Autodesk Fusion 360 part; units mm, degrees
(part 10 of 14)
  arc A2922 (59.8678, 11.2776) -> (59.8678, 11.7856) centre (59.8678, 11.5316) ccw
  line L4390 (48.7934, 56.1848) -> (48.1838, 56.1848)
  line L4391 (62.1538, 11.5316) -> (62.6618, 11.5316)
  arc A2923 (62.4078, 11.1379) -> (62.4078, 11.9253) centre (62.4078, 11.5316) ccw
  arc A2924 (62.4078, 11.9253) -> (62.4078, 11.1379) centre (62.4078, 11.5316) ccw
  line L4392 (62.4078, 11.2776) -> (62.4078, 11.7856)
  arc A2925 (62.4078, 11.9253) -> (62.4078, 11.1379) centre (62.4078, 11.5316) ccw
  arc A2926 (48.26, 58.6184) -> (48.26, 58.5168) centre (48.26, 58.5676) ccw
  line L4393 (48.9712, 60.833) -> (48.006, 60.833)
  arc A2927 (62.1602, 11.5316) -> (62.6555, 11.5316) centre (62.4078, 11.5316) ccw
  line L4394 (48.26, 58.5676) -> (48.768, 58.5676)
  line L4395 (48.1838, 57.2008) -> (48.7934, 57.2008)
  line L4396 (48.1838, 56.1848) -> (48.1838, 57.2008)
  line L4397 (48.7934, 56.1848) -> (48.1838, 56.1848)
  arc A2928 (59.8678, 11.7856) -> (59.8678, 11.2776) centre (59.8678, 11.5316) ccw
  line L4398 (62.4078, 11.2776) -> (62.4078, 11.7856)
  line L4399 (48.9712, 59.1566) -> (48.9712, 60.833)
  line L4400 (48.1838, 56.1848) -> (48.1838, 57.2008)
  arc A2929 (62.4078, 11.9253) -> (62.4078, 11.1379) centre (62.4078, 11.5316) ccw
  line L4401 (48.9386, 60.6948) -> (48.0386, 60.6948)
  arc A2930 (48.26, 58.5168) -> (48.26, 58.6184) centre (48.26, 58.5676) ccw
  arc A2931 (59.8678, 11.9253) -> (59.8678, 11.1379) centre (59.8678, 11.5316) ccw
  line L4402 (77.1398, 33.401) -> (76.5302, 33.401)
  arc A2932 (48.768, 58.0088) -> (48.768, 58.1104) centre (48.768, 58.0596) ccw
  line L4403 (48.9386, 60.6948) -> (48.0386, 60.6948)
  line L4404 (48.768, 58.0596) -> (48.26, 58.0596)
  line L4405 (76.2508, 33.784) -> (76.2508, 34.034)
  line L4406 (75.646, 34.459) -> (75.646, 33.359)
  line L4407 (48.9712, 60.833) -> (48.006, 60.833)
  line L4408 (41.36, 55.926) -> (41.36, 55.326)
  line L4409 (41.402, 55.3212) -> (41.402, 55.9308)
  line L4410 (76.2508, 34.034) -> (75.6412, 34.034)
  line L4411 (42.46, 55.326) -> (42.46, 55.926)
  line L4412 (75.6412, 34.034) -> (75.6412, 33.784)
  line L4413 (41.785, 60.5028) -> (41.785, 59.8932)
  line L4414 (48.9712, 59.1566) -> (48.9712, 60.833)
  line L4415 (76.5302, 34.417) -> (77.1398, 34.417)
  line L4416 (75.6412, 34.417) -> (76.2508, 34.417)
  arc A2933 (48.514, 58.0088) -> (48.514, 58.1104) centre (48.514, 58.0596) ccw
  line L4417 (77.135, 33.359) -> (77.135, 34.459)
  line L4418 (48.7934, 57.2008) -> (48.7934, 56.1848)
  line L4419 (48.514, 58.0596) -> (48.26, 58.5676)
  line L4420 (75.646, 33.359) -> (76.246, 33.359)
  line L4421 (76.535, 34.459) -> (76.535, 33.359)
  line L4422 (75.6412, 33.784) -> (76.2508, 33.784)
  line L4423 (75.6412, 33.401) -> (75.6412, 34.417)
  line L4424 (77.1398, 34.417) -> (77.1398, 33.401)
  line L4425 (77.1398, 33.401) -> (76.5302, 33.401)
  line L4426 (41.402, 60.5028) -> (42.418, 60.5028)
  line L4427 (42.035, 60.5028) -> (41.785, 60.5028)
  line L4428 (42.46, 59.898) -> (42.46, 60.498)
  line L4429 (42.418, 59.8932) -> (41.402, 59.8932)
  line L4430 (48.006, 59.1566) -> (48.9712, 59.1566)
  line L4431 (48.7886, 56.1428) -> (48.7886, 57.2428)
  line L4432 (48.1886, 57.2428) -> (48.1886, 56.1428)
  line L4433 (48.7934, 57.2008) -> (48.7934, 56.1848)
  arc A2934 (48.514, 58.1104) -> (48.514, 58.0088) centre (48.514, 58.0596) ccw
  line L4434 (76.5302, 33.784) -> (77.1398, 33.784)
  line L4435 (76.535, 33.359) -> (77.135, 33.359)
  line L4436 (76.246, 33.359) -> (76.246, 34.459)
  line L4437 (42.418, 60.5028) -> (42.418, 59.8932)
  line L4438 (42.418, 55.9308) -> (42.418, 55.3212)
  line L4439 (41.402, 59.8932) -> (41.402, 60.5028)
  line L4440 (41.402, 60.5028) -> (42.418, 60.5028)
  line L4441 (48.7886, 57.2428) -> (48.1886, 57.2428)
  line L4442 (76.2508, 33.401) -> (75.6412, 33.401)
  arc A2935 (48.768, 58.5168) -> (48.768, 58.6184) centre (48.768, 58.5676) ccw
  line L4443 (42.418, 59.8932) -> (41.402, 59.8932)
  line L4444 (48.9386, 59.2948) -> (48.0386, 59.2948)
  arc A2936 (48.768, 58.1104) -> (48.768, 58.0088) centre (48.768, 58.0596) ccw
  line L4445 (76.2508, 34.417) -> (76.2508, 33.401)
  line L4446 (76.5302, 33.401) -> (76.5302, 34.417)
  line L4447 (48.7934, 56.8178) -> (48.1838, 56.8178)
  line L4448 (76.246, 34.459) -> (75.646, 34.459)
  line L4449 (76.2508, 33.401) -> (75.6412, 33.401)
  line L4450 (41.402, 55.3212) -> (41.402, 55.9308)
  line L4451 (41.36, 55.326) -> (42.46, 55.326)
  line L4452 (41.785, 59.8932) -> (42.035, 59.8932)
  line L4453 (48.768, 58.5676) -> (48.514, 58.0596)
  line L4454 (75.6412, 33.401) -> (75.6412, 34.417)
  line L4455 (42.418, 55.3212) -> (41.402, 55.3212)
  line L4456 (77.135, 34.459) -> (76.535, 34.459)
  arc A2937 (48.768, 58.6184) -> (48.768, 58.5168) centre (48.768, 58.5676) ccw
  line L4457 (76.5302, 34.417) -> (77.1398, 34.417)
  line L4458 (41.785, 55.3212) -> (42.035, 55.3212)
  line L4459 (42.46, 55.926) -> (41.36, 55.926)
  line L4460 (74.041, 34.5948) -> (74.041, 33.9852)
  line L4461 (74.041, 34.8742) -> (73.025, 34.8742)
  line L4462 (73.025, 34.5948) -> (74.041, 34.5948)
  line L4463 (72.983, 34.879) -> (74.083, 34.879)
  line L4464 (73.658, 34.8742) -> (73.658, 35.4838)
  line L4465 (77.2668, 19.304) -> (76.6572, 19.304)
  line L4466 (76.6572, 19.937) -> (76.6572, 19.687)
  line L4467 (77.262, 20.362) -> (76.662, 20.362)
  line L4468 (74.083, 35.479) -> (72.983, 35.479)
  line L4469 (42.035, 59.8932) -> (42.035, 60.5028)
  line L4470 (74.041, 33.9852) -> (73.025, 33.9852)
  line L4471 (74.083, 34.879) -> (74.083, 35.479)
  line L4472 (72.983, 34.59) -> (72.983, 33.99)
  line L4473 (73.658, 34.5948) -> (73.408, 34.5948)
  line L4474 (73.408, 33.9852) -> (73.658, 33.9852)
  line L4475 (77.262, 19.262) -> (77.262, 20.362)
  line L4476 (76.5302, 33.401) -> (76.5302, 34.417)
  line L4477 (76.6572, 19.304) -> (76.6572, 20.32)
  line L4478 (73.025, 33.9852) -> (73.025, 34.5948)
  line L4479 (74.041, 34.8742) -> (73.025, 34.8742)
  line L4480 (74.083, 33.99) -> (74.083, 34.59)
  line L4481 (73.025, 35.4838) -> (74.041, 35.4838)
  line L4482 (73.025, 35.4838) -> (74.041, 35.4838)
  line L4483 (74.083, 34.59) -> (72.983, 34.59)
  line L4484 (73.408, 34.5948) -> (73.408, 33.9852)
  line L4485 (77.2668, 19.937) -> (76.6572, 19.937)
  line L4486 (76.6572, 19.304) -> (76.6572, 20.32)
  line L4487 (74.041, 34.5948) -> (74.041, 33.9852)
  line L4488 (76.6572, 20.32) -> (77.2668, 20.32)
  line L4489 (73.408, 35.4838) -> (73.408, 34.8742)
  line L4490 (76.662, 19.262) -> (77.262, 19.262)
  line L4491 (74.041, 33.9852) -> (73.025, 33.9852)
  line L4492 (74.041, 35.4838) -> (74.041, 34.8742)
  line L4493 (76.6572, 20.32) -> (77.2668, 20.32)
  line L4494 (75.6412, 34.417) -> (76.2508, 34.417)
  line L4495 (76.662, 20.362) -> (76.662, 19.262)
  line L4496 (76.5302, 34.034) -> (76.5302, 33.784)
  line L4497 (74.041, 35.4838) -> (74.041, 34.8742)
  line L4498 (77.2668, 20.32) -> (77.2668, 19.304)
  line L4499 (77.1398, 33.784) -> (77.1398, 34.034)
  line L4500 (41.402, 55.9308) -> (42.418, 55.9308)
  line L4501 (77.1398, 34.034) -> (76.5302, 34.034)
  line L4502 (42.035, 55.3212) -> (42.035, 55.9308)
  line L4503 (42.418, 55.3212) -> (41.402, 55.3212)
  line L4504 (41.785, 55.9308) -> (41.785, 55.3212)
  line L4505 (73.025, 34.5948) -> (74.041, 34.5948)
  line L4506 (77.1398, 34.417) -> (77.1398, 33.401)
  line L4507 (73.408, 34.8742) -> (73.658, 34.8742)
  line L4508 (41.402, 59.8932) -> (41.402, 60.5028)
  line L4509 (73.025, 33.9852) -> (73.025, 34.5948)
  line L4510 (42.418, 55.9308) -> (42.418, 55.3212)
  line L4511 (42.035, 55.9308) -> (41.785, 55.9308)
  line L4512 (76.2508, 34.417) -> (76.2508, 33.401)
  line L4513 (77.2668, 19.687) -> (77.2668, 19.937)
  line L4514 (72.983, 33.99) -> (74.083, 33.99)
  line L4515 (73.658, 35.4838) -> (73.408, 35.4838)
  line L4516 (41.402, 55.9308) -> (42.418, 55.9308)
  line L4517 (73.025, 34.8742) -> (73.025, 35.4838)
  line L4518 (72.983, 35.479) -> (72.983, 34.879)
  line L4519 (76.6572, 19.687) -> (77.2668, 19.687)
  line L4520 (77.2668, 19.304) -> (76.6572, 19.304)
  line L4521 (77.2668, 20.32) -> (77.2668, 19.304)
  line L4522 (73.658, 33.9852) -> (73.658, 34.5948)
  line L4523 (73.025, 34.8742) -> (73.025, 35.4838)
  line L4524 (61.849, 59.309) -> (61.849, 61.849)
  line L4525 (73.025, 19.2278) -> (74.041, 19.2278)
  line L4526 (59.5884, 59.5884) -> (61.5696, 59.5884)
  line L4527 (61.5696, 59.5884) -> (61.5696, 61.5696)
  line L4528 (76.3778, 20.32) -> (76.3778, 19.304)
  line L4529 (72.983, 19.512) -> (74.083, 19.512)
  line L4530 (75.7682, 20.32) -> (76.3778, 20.32)
  line L4531 (61.849, 61.849) -> (59.309, 61.849)
  line L4532 (73.408, 20.1168) -> (73.408, 19.5072)
  line L4533 (75.773, 20.362) -> (75.773, 19.262)
  line L4534 (74.041, 18.6182) -> (73.025, 18.6182)
  line L4535 (73.408, 18.6182) -> (73.658, 18.6182)
  line L4536 (72.983, 19.223) -> (72.983, 18.623)
  line L4537 (73.658, 18.6182) -> (73.658, 19.2278)
  line L4538 (76.373, 20.362) -> (75.773, 20.362)
  line L4539 (74.083, 20.112) -> (72.983, 20.112)
  line L4540 (73.025, 20.1168) -> (74.041, 20.1168)
  line L4541 (59.309, 59.944) -> (59.944, 59.309)
  line L4542 (59.944, 59.309) -> (61.849, 59.309)
  line L4543 (59.5884, 61.5696) -> (59.5884, 59.5884)
  line L4544 (66.3956, 61.5696) -> (64.4144, 61.5696)
  line L4545 (73.025, 18.6182) -> (73.025, 19.2278)
  line L4546 (72.983, 20.112) -> (72.983, 19.512)
  line L4547 (75.773, 19.262) -> (76.373, 19.262)
  line L4548 (74.041, 20.1168) -> (74.041, 19.5072)
  line L4549 (75.7682, 20.32) -> (76.3778, 20.32)
  line L4550 (62.0776, 59.4741) -> (62.0776, 61.6839)
  line L4551 (66.675, 61.849) -> (64.135, 61.849)
  line L4552 (66.675, 59.309) -> (66.675, 61.849)
  line L4553 (59.0804, 59.4741) -> (59.0804, 61.6839)
  line L4554 (64.135, 61.849) -> (64.135, 59.944)
  line L4555 (73.658, 19.5072) -> (73.658, 20.1168)
  line L4556 (74.083, 19.223) -> (72.983, 19.223)
  line L4557 (75.7682, 19.304) -> (75.7682, 20.32)
  line L4558 (73.658, 20.1168) -> (73.408, 20.1168)
  line L4559 (72.983, 18.623) -> (74.083, 18.623)
  line L4560 (76.3778, 19.687) -> (76.3778, 19.937)
  line L4561 (75.7682, 19.304) -> (75.7682, 20.32)
  line L4562 (62.0776, 59.4741) -> (62.0776, 61.6839)
  line L4563 (59.309, 61.849) -> (59.309, 59.944)
  line L4564 (75.7682, 19.937) -> (75.7682, 19.687)
  line L4565 (73.408, 19.2278) -> (73.408, 18.6182)
  line L4566 (74.083, 19.512) -> (74.083, 20.112)
  line L4567 (76.373, 19.262) -> (76.373, 20.362)
  line L4568 (73.025, 18.6182) -> (73.025, 19.2278)
  line L4569 (74.041, 20.1168) -> (74.041, 19.5072)
  line L4570 (74.041, 19.2278) -> (74.041, 18.6182)
  line L4571 (76.3778, 19.937) -> (75.7682, 19.937)
  line L4572 (75.7682, 19.687) -> (76.3778, 19.687)
  line L4573 (74.041, 19.5072) -> (73.025, 19.5072)
  line L4574 (73.658, 19.2278) -> (73.408, 19.2278)
  line L4575 (73.025, 19.5072) -> (73.025, 20.1168)
  line L4576 (74.041, 19.2278) -> (74.041, 18.6182)
  line L4577 (76.3778, 19.304) -> (75.7682, 19.304)
  line L4578 (61.5696, 61.5696) -> (59.5884, 61.5696)
  line L4579 (76.3778, 20.32) -> (76.3778, 19.304)
  line L4580 (74.083, 18.623) -> (74.083, 19.223)
  line L4581 (73.025, 20.1168) -> (74.041, 20.1168)
  line L4582 (73.025, 19.2278) -> (74.041, 19.2278)
  line L4583 (76.3778, 19.304) -> (75.7682, 19.304)
  line L4584 (74.041, 19.5072) -> (73.025, 19.5072)
  line L4585 (73.025, 19.5072) -> (73.025, 20.1168)
  line L4586 (74.041, 18.6182) -> (73.025, 18.6182)
  line L4587 (73.408, 19.5072) -> (73.658, 19.5072)
  line L4588 (84.917, 57.362) -> (85.517, 57.362)
  line L4589 (22.733, 53.1368) -> (22.733, 49.7332)
  line L4590 (85.517, 57.362) -> (85.517, 58.462)
  line L4591 (84.9122, 58.42) -> (85.5218, 58.42)
  line L4592 (26.455, 42.675) -> (28.155, 42.675)
  line L4593 (60.071, 59.0804) -> (61.087, 59.0804)
  line L4594 (66.9036, 59.4741) -> (66.9036, 61.6839)
  line L4595 (26.455, 39.875) -> (28.155, 39.875)
  line L4596 (28.205, 42.975) -> (26.405, 42.975)
  line L4597 (26.405, 39.575) -> (28.205, 39.575)
  line L4598 (60.071, 62.0776) -> (61.087, 62.0776)
  line L4599 (28.194, 42.9768) -> (26.416, 42.9768)
  line L4600 (84.9122, 58.42) -> (85.5218, 58.42)
  line L4601 (85.517, 58.462) -> (84.917, 58.462)
  line L4602 (28.194, 42.9768) -> (26.416, 42.9768)
  line L4603 (63.9064, 59.4741) -> (63.9064, 61.6839)
  line L4604 (26.416, 39.5732) -> (28.194, 39.5732)
  line L4605 (64.897, 62.0776) -> (65.913, 62.0776)
  line L4606 (63.9064, 59.4741) -> (63.9064, 61.6839)
  line L4607 (84.9122, 57.404) -> (84.9122, 58.42)
  line L4608 (24.522, 49.735) -> (24.522, 53.135)
  line L4609 (64.4144, 61.5696) -> (64.4144, 59.5884)
  line L4610 (66.9036, 59.4741) -> (66.9036, 61.6839)
  line L4611 (85.5218, 58.42) -> (85.5218, 57.404)
  line L4612 (28.194, 39.5732) -> (28.194, 42.9768)
  line L4613 (24.511, 49.7332) -> (24.511, 53.1368)
  line L4614 (22.722, 53.135) -> (22.722, 49.735)
  line L4615 (24.511, 53.1368) -> (22.733, 53.1368)
  line L4616 (60.071, 59.0804) -> (61.087, 59.0804)
  line L4617 (26.416, 42.9768) -> (26.416, 39.5732)
  line L4618 (85.5218, 58.037) -> (84.9122, 58.037)
  line L4619 (22.733, 53.1368) -> (22.733, 49.7332)
  line L4620 (22.733, 49.7332) -> (24.511, 49.7332)
  line L4621 (22.733, 49.7332) -> (24.511, 49.7332)
  line L4622 (84.9122, 57.404) -> (84.9122, 58.42)
  line L4623 (59.0804, 59.4741) -> (59.0804, 61.6839)
  line L4624 (66.9036, 59.4741) -> (66.9036, 61.6839)
  line L4625 (26.455, 42.675) -> (28.155, 42.675)
  line L4626 (22.722, 49.735) -> (24.522, 49.735)
  line L4627 (64.897, 59.0804) -> (65.913, 59.0804)
  line L4628 (64.897, 59.0804) -> (65.913, 59.0804)
  line L4629 (59.0804, 59.4741) -> (59.0804, 61.6839)
  line L4630 (64.897, 62.0776) -> (65.913, 62.0776)
  line L4631 (62.0776, 59.4741) -> (62.0776, 61.6839)
  line L4632 (60.071, 62.0776) -> (61.087, 62.0776)
  line L4633 (64.135, 59.944) -> (64.77, 59.309)
  line L4634 (66.3956, 59.5884) -> (66.3956, 61.5696)
  line L4635 (64.77, 59.309) -> (66.675, 59.309)
  line L4636 (60.071, 62.0776) -> (61.087, 62.0776)
  line L4637 (60.071, 59.0804) -> (61.087, 59.0804)
  line L4638 (64.4144, 59.5884) -> (66.3956, 59.5884)
  line L4639 (28.205, 39.575) -> (28.205, 42.975)
  line L4640 (64.897, 59.0804) -> (65.913, 59.0804)
  line L4641 (85.5218, 57.404) -> (84.9122, 57.404)
  line L4642 (84.9122, 57.787) -> (85.5218, 57.787)
  line L4643 (64.897, 62.0776) -> (65.913, 62.0776)
  line L4644 (28.194, 39.5732) -> (28.194, 42.9768)
  line L4645 (26.455, 39.875) -> (28.155, 39.875)
  line L4646 (84.9122, 58.037) -> (84.9122, 57.787)
  line L4647 (24.511, 49.7332) -> (24.511, 53.1368)
  line L4648 (85.5218, 58.42) -> (85.5218, 57.404)
  line L4649 (26.416, 42.9768) -> (26.416, 39.5732)
  line L4650 (63.9064, 59.4741) -> (63.9064, 61.6839)
  line L4651 (26.416, 39.5732) -> (28.194, 39.5732)
  line L4652 (74.589, 2.579) -> (73.239, 2.579)
  line L4653 (68.1482, 2.286) -> (68.1482, 4.572)
  line L4654 (22.772, 52.835) -> (24.472, 52.835)
  line L4655 (86.106, 52.1208) -> (86.106, 53.5432)
  line L4656 (83.863, 53.557) -> (83.863, 52.107)
  line L4657 (66.712, 4.529) -> (66.712, 2.329)
  line L4658 (24.511, 53.1368) -> (22.733, 53.1368)
  line L4659 (68.1482, 2.286) -> (68.1482, 4.572)
  line L4660 (86.106, 53.5432) -> (83.82, 53.5432)
  line L4661 (83.399, 56.095) -> (84.749, 56.095)
  line L4662 (83.399, 56.095) -> (84.749, 56.095)
  line L4663 (73.189, 4.529) -> (73.189, 2.329)
  line L4664 (83.82, 52.1208) -> (86.106, 52.1208)
  line L4665 (22.772, 52.835) -> (24.472, 52.835)
  line L4666 (66.762, 4.279) -> (68.112, 4.279)
  line L4667 (73.2028, 4.572) -> (73.2028, 2.286)
  line L4668 (66.762, 4.279) -> (68.112, 4.279)
  line L4669 (84.113, 53.507) -> (84.113, 52.157)
  line L4670 (22.772, 50.035) -> (24.472, 50.035)
  line L4671 (85.813, 53.507) -> (85.813, 52.157)
  line L4672 (66.762, 2.579) -> (68.112, 2.579)
  line L4673 (85.5218, 57.404) -> (84.9122, 57.404)
  line L4674 (66.712, 2.329) -> (68.162, 2.329)
  line L4675 (74.639, 2.329) -> (74.639, 4.529)
  line L4676 (22.772, 50.035) -> (24.472, 50.035)
  line L4677 (84.7852, 54.102) -> (84.7852, 56.388)
  line L4678 (86.063, 52.107) -> (86.063, 53.557)
  line L4679 (84.7852, 56.388) -> (83.3628, 56.388)
  line L4680 (68.162, 2.329) -> (68.162, 4.529)
  line L4681 (73.2028, 2.286) -> (74.6252, 2.286)
  line L4682 (66.7258, 2.286) -> (68.1482, 2.286)
  line L4683 (74.6252, 2.286) -> (74.6252, 4.572)
  line L4684 (83.82, 52.1208) -> (86.106, 52.1208)
  line L4685 (74.589, 2.579) -> (73.239, 2.579)
  line L4686 (66.7258, 2.286) -> (68.1482, 2.286)
  line L4687 (73.2028, 2.286) -> (74.6252, 2.286)
  line L4688 (68.1482, 4.572) -> (66.7258, 4.572)
  line L4689 (68.162, 4.529) -> (66.712, 4.529)
  line L4690 (66.762, 4.279) -> (68.112, 4.279)
  line L4691 (84.917, 58.462) -> (84.917, 57.362)
  line L4692 (26.405, 42.975) -> (26.405, 39.575)
  line L4693 (24.522, 53.135) -> (22.722, 53.135)
  line L4694 (74.639, 4.529) -> (73.189, 4.529)
  line L4695 (26.455, 42.675) -> (28.155, 42.675)
  line L4696 (66.7258, 4.572) -> (66.7258, 2.286)
  line L4697 (22.772, 50.035) -> (24.472, 50.035)
  line L4698 (66.7258, 4.572) -> (66.7258, 2.286)
  line L4699 (74.6252, 2.286) -> (74.6252, 4.572)
  line L4700 (74.6252, 4.572) -> (73.2028, 4.572)
  line L4701 (85.5218, 57.787) -> (85.5218, 58.037)
  line L4702 (68.1482, 4.572) -> (66.7258, 4.572)
  line L4703 (73.189, 2.329) -> (74.639, 2.329)
  line L4704 (26.455, 39.875) -> (28.155, 39.875)
  line L4705 (73.2028, 4.572) -> (73.2028, 2.286)
  line L4706 (66.762, 2.579) -> (68.112, 2.579)
  line L4707 (84.7852, 56.388) -> (83.3628, 56.388)
  line L4708 (83.399, 54.395) -> (84.749, 54.395)
  line L4709 (83.399, 54.395) -> (84.749, 54.395)
  line L4710 (74.6252, 4.572) -> (73.2028, 4.572)
  line L4711 (74.589, 4.279) -> (73.239, 4.279)
  line L4712 (22.772, 52.835) -> (24.472, 52.835)
  line L4713 (83.399, 54.395) -> (84.749, 54.395)
  line L4714 (66.762, 2.579) -> (68.112, 2.579)
  line L4715 (74.589, 2.579) -> (73.239, 2.579)
  line L4716 (27.85, 58.844) -> (29.3, 58.844)
  line L4717 (84.799, 54.145) -> (84.799, 56.345)
  line L4718 (83.399, 56.095) -> (84.749, 56.095)
  line L4719 (83.3628, 56.388) -> (83.3628, 54.102)
  line L4720 (32.385, 32.5628) -> (32.385, 33.9852)
  line L4721 (32.385, 33.9852) -> (30.099, 33.9852)
  line L4722 (83.863, 52.107) -> (86.063, 52.107)
  line L4723 (32.342, 36.666) -> (30.142, 36.666)
  line L4724 (32.342, 35.216) -> (32.342, 36.666)
  line L4725 (32.092, 33.949) -> (32.092, 32.599)
  line L4726 (83.3628, 56.388) -> (83.3628, 54.102)
  line L4727 (29.3, 61.044) -> (27.85, 61.044)
  line L4728 (84.113, 53.507) -> (84.113, 52.157)
  line L4729 (30.142, 35.216) -> (32.342, 35.216)
  line L4730 (27.8638, 58.801) -> (29.2862, 58.801)
  line L4731 (30.099, 33.9852) -> (30.099, 32.5628)
  line L4732 (83.349, 54.145) -> (84.799, 54.145)
  line L4733 (29.2862, 61.087) -> (27.8638, 61.087)
  line L4734 (74.589, 4.279) -> (73.239, 4.279)
  line L4735 (85.813, 53.507) -> (85.813, 52.157)
  line L4736 (30.099, 35.2298) -> (32.385, 35.2298)
  line L4737 (32.385, 36.6522) -> (30.099, 36.6522)
  line L4738 (32.092, 36.616) -> (32.092, 35.266)
  line L4739 (27.85, 61.044) -> (27.85, 58.844)
  line L4740 (29.3, 58.844) -> (29.3, 61.044)
  line L4741 (30.142, 36.666) -> (30.142, 35.216)
  line L4742 (30.099, 33.9852) -> (30.099, 32.5628)
  line L4743 (30.392, 33.949) -> (30.392, 32.599)
  line L4744 (84.799, 56.345) -> (83.349, 56.345)
  line L4745 (84.113, 53.507) -> (84.113, 52.157)
  line L4746 (85.813, 53.507) -> (85.813, 52.157)
  line L4747 (83.82, 53.5432) -> (83.82, 52.1208)
  line L4748 (32.342, 33.999) -> (30.142, 33.999)
  line L4749 (32.342, 32.549) -> (32.342, 33.999)
  line L4750 (32.385, 36.6522) -> (30.099, 36.6522)
  line L4751 (86.106, 53.5432) -> (83.82, 53.5432)
  line L4752 (30.392, 36.616) -> (30.392, 35.266)
  line L4753 (32.385, 32.5628) -> (32.385, 33.9852)
  line L4754 (86.063, 53.557) -> (83.863, 53.557)
  line L4755 (30.099, 32.5628) -> (32.385, 32.5628)
  line L4756 (83.82, 53.5432) -> (83.82, 52.1208)
  line L4757 (74.589, 4.279) -> (73.239, 4.279)
  line L4758 (30.099, 32.5628) -> (32.385, 32.5628)
  line L4759 (32.385, 33.9852) -> (30.099, 33.9852)
  line L4760 (84.7852, 54.102) -> (84.7852, 56.388)
  line L4761 (32.092, 36.616) -> (32.092, 35.266)
  line L4762 (27.8638, 61.087) -> (27.8638, 58.801)
  line L4763 (30.099, 35.2298) -> (32.385, 35.2298)
  line L4764 (32.092, 33.949) -> (32.092, 32.599)
  line L4765 (30.142, 32.549) -> (32.342, 32.549)
  line L4766 (30.392, 33.949) -> (30.392, 32.599)
  line L4767 (83.3628, 54.102) -> (84.7852, 54.102)
  line L4768 (27.8638, 61.087) -> (27.8638, 58.801)
  line L4769 (30.099, 36.6522) -> (30.099, 35.2298)
  line L4770 (30.392, 36.616) -> (30.392, 35.266)
  line L4771 (32.092, 36.616) -> (32.092, 35.266)
  line L4772 (86.106, 52.1208) -> (86.106, 53.5432)
  line L4773 (30.392, 33.949) -> (30.392, 32.599)
  line L4774 (30.392, 36.616) -> (30.392, 35.266)
  line L4775 (29.2862, 58.801) -> (29.2862, 61.087)
  line L4776 (83.3628, 54.102) -> (84.7852, 54.102)
  line L4777 (32.385, 35.2298) -> (32.385, 36.6522)
  line L4778 (83.349, 56.345) -> (83.349, 54.145)
  line L4779 (30.142, 33.999) -> (30.142, 32.549)
  line L4780 (32.092, 33.949) -> (32.092, 32.599)
  line L4781 (29.805, 61.81) -> (31.155, 61.81)
  line L4782 (29.7688, 59.817) -> (31.1912, 59.817)
  arc A2938 (64.897, 52.04) -> (64.897, 52.608) centre (64.897, 52.324) ccw
  line L4783 (66.3067, 54.098) -> (65.4177, 54.098)
  line L4784 (66.3067, 55.098) -> (65.4177, 55.098)
  line L4785 (29.7688, 59.817) -> (31.1912, 59.817)
  line L4786 (65.4558, 51.308) -> (60.833, 51.308)
  line L4787 (66.3067, 54.098) -> (65.4177, 54.098)
  line L4788 (66.3067, 55.598) -> (65.4177, 55.598)
  line L4789 (65.123, 55.8927) -> (65.123, 56.7817)
  line L4790 (31.205, 59.86) -> (31.205, 62.06)
  line L4791 (29.805, 60.11) -> (31.155, 60.11)
  line L4792 (31.1912, 62.103) -> (29.7688, 62.103)
  line L4793 (31.1912, 59.817) -> (31.1912, 62.103)
  line L4794 (66.3067, 55.598) -> (65.4177, 55.598)
  line L4795 (29.805, 60.11) -> (31.155, 60.11)
  line L4796 (66.3067, 52.098) -> (65.4177, 52.098)
  line L4797 (27.9, 60.794) -> (29.25, 60.794)
  line L4798 (66.3067, 52.098) -> (65.4177, 52.098)
  line L4799 (29.7688, 62.103) -> (29.7688, 59.817)
  line L4800 (66.3067, 54.598) -> (65.4177, 54.598)
  line L4801 (66.3067, 52.598) -> (65.4177, 52.598)
  line L4802 (66.3067, 54.098) -> (65.4177, 54.098)
  line L4803 (66.3067, 54.598) -> (65.4177, 54.598)
  line L4804 (66.3067, 54.598) -> (65.4177, 54.598)
  line L4805 (29.7688, 62.103) -> (29.7688, 59.817)
  line L4806 (66.3067, 53.598) -> (65.4177, 53.598)
  line L4807 (66.3067, 52.098) -> (65.4177, 52.098)
  line L4808 (60.833, 56.388) -> (65.913, 56.388)
  line L4809 (60.833, 51.308) -> (60.833, 56.388)
  line L4810 (27.8638, 58.801) -> (29.2862, 58.801)
  line L4811 (29.805, 60.11) -> (31.155, 60.11)
  line L4812 (65.913, 51.7652) -> (65.4558, 51.308)
  line L4813 (29.2862, 61.087) -> (27.8638, 61.087)
  line L4814 (31.205, 62.06) -> (29.755, 62.06)
  line L4815 (30.099, 36.6522) -> (30.099, 35.2298)
  line L4816 (27.9, 60.794) -> (29.25, 60.794)
  line L4817 (31.1912, 59.817) -> (31.1912, 62.103)
  line L4818 (27.9, 59.094) -> (29.25, 59.094)
  line L4819 (66.3067, 55.098) -> (65.4177, 55.098)
  line L4820 (66.3067, 52.598) -> (65.4177, 52.598)
  line L4821 (29.755, 59.86) -> (31.205, 59.86)
  line L4822 (32.385, 35.2298) -> (32.385, 36.6522)
  arc A2939 (64.897, 52.608) -> (64.897, 52.04) centre (64.897, 52.324) ccw
  line L4823 (65.913, 56.388) -> (65.913, 51.7652)
  arc A2940 (66.597, 51.808) -> (66.597, 51.24) centre (66.597, 51.524) ccw
  line L4824 (66.3067, 53.598) -> (65.4177, 53.598)
  line L4825 (66.3067, 52.598) -> (65.4177, 52.598)
  line L4826 (29.805, 61.81) -> (31.155, 61.81)
  line L4827 (31.1912, 62.103) -> (29.7688, 62.103)
  line L4828 (27.9, 59.094) -> (29.25, 59.094)
  line L4829 (66.3067, 55.098) -> (65.4177, 55.098)
  line L4830 (66.3067, 53.098) -> (65.4177, 53.098)
  line L4831 (27.9, 60.794) -> (29.25, 60.794)
  line L4832 (29.755, 62.06) -> (29.755, 59.86)
  arc A2941 (66.597, 51.24) -> (66.597, 51.808) centre (66.597, 51.524) ccw
  line L4833 (29.2862, 58.801) -> (29.2862, 61.087)
  line L4834 (29.805, 61.81) -> (31.155, 61.81)
  line L4835 (27.9, 59.094) -> (29.25, 59.094)
  line L4836 (66.3067, 53.098) -> (65.4177, 53.098)
  line L4837 (66.3067, 53.098) -> (65.4177, 53.098)
  line L4838 (66.3067, 55.598) -> (65.4177, 55.598)
  line L4839 (66.3067, 53.598) -> (65.4177, 53.598)
  line L4840 (21.9227, 8.9205) -> (21.9227, 9.5301)
  line L4841 (22.3058, 9.5301) -> (22.3058, 8.9205)
  line L4842 (63.373, 52.7488) -> (63.373, 55.0488)
  line L4843 (22.3058, 8.9205) -> (22.5557, 8.9205)
  line L4844 (22.5557, 9.5301) -> (22.3058, 9.5301)
  line L4845 (61.3283, 54.598) -> (60.4393, 54.598)
  line L4846 (21.9227, 9.5301) -> (22.9387, 9.5301)
  line L4847 (63.373, 52.7488) -> (63.373, 55.0488)
  line L4848 (22.5557, 8.9205) -> (22.5557, 9.5301)
  line L4849 (22.9807, 9.5253) -> (21.8807, 9.5253)
  line L4850 (61.3283, 53.598) -> (60.4393, 53.598)
  line L4851 (61.623, 50.9143) -> (61.623, 51.8033)
  line L4852 (61.3283, 52.598) -> (60.4393, 52.598)
  line L4853 (65.123, 50.9143) -> (65.123, 51.8033)
  line L4854 (63.123, 50.9143) -> (63.123, 51.8033)
  line L4855 (62.623, 50.9143) -> (62.623, 51.8033)
  line L4856 (61.3283, 53.098) -> (60.4393, 53.098)
  line L4857 (61.3283, 54.598) -> (60.4393, 54.598)
  line L4858 (61.623, 50.9143) -> (61.623, 51.8033)
  line L4859 (62.123, 50.9143) -> (62.123, 51.8033)
  line L4860 (65.123, 50.9143) -> (65.123, 51.8033)
  line L4861 (61.3283, 53.098) -> (60.4393, 53.098)
  line L4862 (61.3283, 53.598) -> (60.4393, 53.598)
  line L4863 (64.123, 50.9143) -> (64.123, 51.8033)
  line L4864 (64.123, 50.9143) -> (64.123, 51.8033)
  line L4865 (22.9387, 8.9205) -> (21.9227, 8.9205)
  line L4866 (61.3283, 52.598) -> (60.4393, 52.598)
  line L4867 (64.123, 50.9143) -> (64.123, 51.8033)
  line L4868 (64.623, 50.9143) -> (64.623, 51.8033)
  line L4869 (21.8807, 8.9253) -> (22.9807, 8.9253)
  line L4870 (61.623, 50.9143) -> (61.623, 51.8033)
  line L4871 (62.123, 50.9143) -> (62.123, 51.8033)
  line L4872 (21.9227, 8.9205) -> (21.9227, 9.5301)
  line L4873 (52.7558, 44.071) -> (52.7558, 44.321)
  line L4874 (63.123, 50.9143) -> (63.123, 51.8033)
  line L4875 (61.3283, 52.598) -> (60.4393, 52.598)
  line L4876 (54.2798, 45.339) -> (54.2798, 44.323)
  line L4877 (52.1462, 44.704) -> (52.7558, 44.704)
  line L4878 (61.3283, 54.098) -> (60.4393, 54.098)
  line L4879 (61.3283, 53.598) -> (60.4393, 53.598)
  line L4880 (63.623, 50.9143) -> (63.623, 51.8033)
  line L4881 (22.9387, 8.9205) -> (21.9227, 8.9205)
  line L4882 (63.123, 50.9143) -> (63.123, 51.8033)
  line L4883 (61.3283, 52.098) -> (60.4393, 52.098)
  line L4884 (61.3283, 54.098) -> (60.4393, 54.098)
  line L4885 (61.3283, 52.098) -> (60.4393, 52.098)
  line L4886 (62.123, 50.9143) -> (62.123, 51.8033)
  line L4887 (63.623, 50.9143) -> (63.623, 51.8033)
  line L4888 (63.623, 50.9143) -> (63.623, 51.8033)
  line L4889 (65.123, 50.9143) -> (65.123, 51.8033)
  line L4890 (63.373, 52.7488) -> (63.373, 55.0488)
  line L4891 (54.2798, 44.956) -> (53.6702, 44.956)
  line L4892 (62.623, 50.9143) -> (62.623, 51.8033)
  line L4893 (21.9227, 9.5301) -> (22.9387, 9.5301)
  line L4894 (64.623, 50.9143) -> (64.623, 51.8033)
  line L4895 (61.3283, 53.098) -> (60.4393, 53.098)
  line L4896 (61.3283, 54.098) -> (60.4393, 54.098)
  line L4897 (22.9807, 8.9253) -> (22.9807, 9.5253)
  line L4898 (64.623, 50.9143) -> (64.623, 51.8033)
  line L4899 (62.623, 50.9143) -> (62.623, 51.8033)
  line L4900 (21.8807, 9.5253) -> (21.8807, 8.9253)
  line L4901 (22.9387, 9.5301) -> (22.9387, 8.9205)
  line L4902 (22.9387, 9.5301) -> (22.9387, 8.9205)
  line L4903 (61.3283, 52.098) -> (60.4393, 52.098)
  line L4904 (60.625, 44.492) -> (60.025, 44.492)
  line L4905 (61.6458, 44.45) -> (61.6458, 43.434)
  line L4906 (61.0362, 43.434) -> (61.0362, 44.45)
  line L4907 (61.0362, 43.817) -> (61.6458, 43.817)
  line L4908 (60.025, 44.492) -> (60.025, 43.392)
  line L4909 (52.751, 44.746) -> (52.151, 44.746)
  line L4910 (60.0202, 43.817) -> (60.6298, 43.817)
  line L4911 (52.7558, 44.321) -> (52.1462, 44.321)
  line L4912 (53.675, 45.381) -> (53.675, 44.281)
  line L4913 (54.2798, 44.323) -> (53.6702, 44.323)
  line L4914 (60.6298, 44.067) -> (60.0202, 44.067)
  line L4915 (52.151, 44.746) -> (52.151, 43.646)
  line L4916 (54.2798, 44.323) -> (53.6702, 44.323)
  line L4917 (67.312, 54.4322) -> (67.562, 54.4322)
  line L4918 (61.041, 43.392) -> (61.641, 43.392)
  line L4919 (60.625, 43.392) -> (60.625, 44.492)
  line L4920 (61.0362, 44.45) -> (61.6458, 44.45)
  line L4921 (52.1462, 44.704) -> (52.7558, 44.704)
  line L4922 (53.6702, 44.956) -> (53.6702, 44.706)
  line L4923 (52.7558, 43.688) -> (52.1462, 43.688)
  line L4924 (68.495, 50.465) -> (67.395, 50.465)
  line L4925 (53.6702, 44.323) -> (53.6702, 45.339)
  line L4926 (52.1462, 43.688) -> (52.1462, 44.704)
  line L4927 (53.6702, 45.339) -> (54.2798, 45.339)
  line L4928 (54.275, 44.281) -> (54.275, 45.381)
  line L4929 (66.929, 54.4322) -> (66.929, 55.0418)
  line L4930 (64.9732, 49.657) -> (65.5828, 49.657)
  line L4931 (65.578, 48.599) -> (65.578, 49.699)
  line L4932 (52.7558, 44.704) -> (52.7558, 43.688)
  line L4933 (61.041, 44.492) -> (61.041, 43.392)
  line L4934 (67.562, 54.1528) -> (67.312, 54.1528)
  line L4935 (67.945, 54.1528) -> (67.945, 53.5432)
  line L4936 (66.929, 53.5432) -> (66.929, 54.1528)
  line L4937 (60.6298, 44.45) -> (60.6298, 43.434)
  line L4938 (66.929, 55.0418) -> (67.945, 55.0418)
  line L4939 (60.6298, 43.434) -> (60.0202, 43.434)
  line L4940 (60.0202, 43.434) -> (60.0202, 44.45)
  line L4941 (52.1462, 44.321) -> (52.1462, 44.071)
  line L4942 (54.275, 45.381) -> (53.675, 45.381)
  line L4943 (60.0202, 44.45) -> (60.6298, 44.45)
  line L4944 (53.6702, 44.706) -> (54.2798, 44.706)
  line L4945 (60.6298, 43.434) -> (60.0202, 43.434)
  line L4946 (60.0202, 44.067) -> (60.0202, 43.817)
  line L4947 (53.6702, 45.339) -> (54.2798, 45.339)
  line L4948 (53.6702, 44.323) -> (53.6702, 45.339)
  line L4949 (54.2798, 45.339) -> (54.2798, 44.323)
  line L4950 (60.6298, 43.817) -> (60.6298, 44.067)
  line L4951 (52.151, 43.646) -> (52.751, 43.646)
  line L4952 (61.6458, 44.45) -> (61.6458, 43.434)
  line L4953 (60.6298, 44.45) -> (60.6298, 43.434)
  line L4954 (61.641, 43.392) -> (61.641, 44.492)
  line L4955 (52.7558, 44.704) -> (52.7558, 43.688)
  line L4956 (53.675, 44.281) -> (54.275, 44.281)
  line L4957 (52.7558, 43.688) -> (52.1462, 43.688)
  line L4958 (52.1462, 44.071) -> (52.7558, 44.071)
  line L4959 (60.0202, 44.45) -> (60.6298, 44.45)
  line L4960 (61.641, 44.492) -> (61.041, 44.492)
  line L4961 (61.6458, 43.434) -> (61.0362, 43.434)
  line L4962 (52.751, 43.646) -> (52.751, 44.746)
  line L4963 (61.0362, 44.45) -> (61.6458, 44.45)
  line L4964 (54.2798, 44.706) -> (54.2798, 44.956)
  line L4965 (52.1462, 43.688) -> (52.1462, 44.704)
  line L4966 (60.0202, 43.434) -> (60.0202, 44.45)
  line L4967 (60.025, 43.392) -> (60.625, 43.392)
  line L4968 (59.4868, 54.61) -> (58.8772, 54.61)
  line L4969 (64.978, 49.699) -> (64.978, 48.599)
  line L4970 (67.945, 54.1528) -> (67.945, 53.5432)
  line L4971 (65.5828, 49.024) -> (65.5828, 49.274)
  line L4972 (67.312, 53.5432) -> (67.562, 53.5432)
  line L4973 (66.887, 54.437) -> (67.987, 54.437)
  line L4974 (66.887, 54.148) -> (66.887, 53.548)
  line L4975 (64.978, 48.599) -> (65.578, 48.599)
  line L4976 (59.482, 55.668) -> (58.882, 55.668)
  line L4977 (63.962, 49.699) -> (63.962, 48.599)
  line L4978 (67.945, 55.0418) -> (67.945, 54.4322)
  line L4979 (64.9732, 48.641) -> (64.9732, 49.657)
  line L4980 (67.945, 53.5432) -> (66.929, 53.5432)
  line L4981 (63.9572, 49.024) -> (64.5668, 49.024)
  line L4982 (68.453, 50.4698) -> (68.453, 49.8602)
  line L4983 (64.9732, 49.274) -> (64.9732, 49.024)
  line L4984 (61.6458, 43.434) -> (61.0362, 43.434)
  line L4985 (67.562, 54.4322) -> (67.562, 55.0418)
  line L4986 (67.987, 53.548) -> (67.987, 54.148)
  line L4987 (61.6458, 43.817) -> (61.6458, 44.067)
  line L4988 (59.4868, 55.626) -> (59.4868, 54.61)
  line L4989 (61.0362, 43.434) -> (61.0362, 44.45)
  line L4990 (67.987, 54.437) -> (67.987, 55.037)
  line L4991 (58.8772, 55.243) -> (58.8772, 54.993)
  line L4992 (59.482, 54.568) -> (59.482, 55.668)
  line L4993 (68.495, 49.865) -> (68.495, 50.465)
  line L4994 (67.562, 53.5432) -> (67.562, 54.1528)
  line L4995 (64.5668, 48.641) -> (63.9572, 48.641)
  line L4996 (58.882, 54.568) -> (59.482, 54.568)
  line L4997 (64.9732, 49.657) -> (65.5828, 49.657)
  line L4998 (67.562, 55.0418) -> (67.312, 55.0418)
  line L4999 (66.929, 54.1528) -> (67.945, 54.1528)
  line L5000 (66.887, 55.037) -> (66.887, 54.437)
  line L5001 (68.453, 49.8602) -> (67.437, 49.8602)
  line L5002 (67.437, 49.8602) -> (67.437, 50.4698)
  line L5003 (67.987, 54.148) -> (66.887, 54.148)
  line L5004 (67.312, 54.1528) -> (67.312, 53.5432)
  line L5005 (64.9732, 49.024) -> (65.5828, 49.024)
  line L5006 (66.929, 54.1528) -> (67.945, 54.1528)
  line L5007 (67.945, 54.4322) -> (66.929, 54.4322)
  line L5008 (66.887, 53.548) -> (67.987, 53.548)
  line L5009 (65.578, 49.699) -> (64.978, 49.699)
  line L5010 (68.07, 49.8602) -> (68.07, 50.4698)
  line L5011 (65.5828, 49.657) -> (65.5828, 48.641)
  line L5012 (65.5828, 48.641) -> (64.9732, 48.641)
  line L5013 (67.395, 50.465) -> (67.395, 49.865)
  line L5014 (61.0362, 44.067) -> (61.0362, 43.817)
  line L5015 (65.5828, 49.274) -> (64.9732, 49.274)
  line L5016 (66.929, 55.0418) -> (67.945, 55.0418)
  line L5017 (65.5828, 48.641) -> (64.9732, 48.641)
  line L5018 (67.312, 55.0418) -> (67.312, 54.4322)
  line L5019 (67.987, 55.037) -> (66.887, 55.037)
  line L5020 (66.929, 54.4322) -> (66.929, 55.0418)
  line L5021 (64.9732, 48.641) -> (64.9732, 49.657)
  line L5022 (67.945, 54.4322) -> (66.929, 54.4322)
  line L5023 (65.5828, 49.657) -> (65.5828, 48.641)
  line L5024 (61.6458, 44.067) -> (61.0362, 44.067)
  line L5025 (67.945, 53.5432) -> (66.929, 53.5432)
  line L5026 (67.945, 55.0418) -> (67.945, 54.4322)
  line L5027 (59.4868, 52.705) -> (58.8772, 52.705)
  line L5028 (64.5668, 49.657) -> (64.5668, 48.641)
  line L5029 (58.8772, 55.626) -> (59.4868, 55.626)
  line L5030 (66.929, 53.5432) -> (66.929, 54.1528)
  line L5031 (59.4868, 54.61) -> (58.8772, 54.61)
  line L5032 (58.882, 52.663) -> (59.482, 52.663)
  line L5033 (67.395, 49.865) -> (68.495, 49.865)
  line L5034 (59.4868, 53.721) -> (59.4868, 52.705)
  line L5035 (64.5668, 49.024) -> (64.5668, 49.274)
  line L5036 (59.4868, 53.088) -> (59.4868, 53.338)
  line L5037 (65.7128, 50.673) -> (65.4629, 50.673)
  line L5038 (65.4629, 50.0634) -> (65.7128, 50.0634)
  line L5039 (59.4868, 53.721) -> (59.4868, 52.705)
  line L5040 (66.0959, 50.0634) -> (65.0799, 50.0634)
  line L5041 (65.0799, 50.673) -> (66.0959, 50.673)
  line L5042 (67.3913, 52.3037) -> (67.3913, 51.2877)
  line L5043 (64.5668, 49.657) -> (64.5668, 48.641)
  line L5044 (58.8772, 53.721) -> (59.4868, 53.721)
  line L5045 (59.482, 53.763) -> (58.882, 53.763)
  line L5046 (67.3913, 52.3037) -> (67.3913, 51.2877)
  line L5047 (67.3913, 51.2877) -> (66.7817, 51.2877)
  line L5048 (59.4868, 55.243) -> (58.8772, 55.243)
  line L5049 (63.9572, 49.274) -> (63.9572, 49.024)
  line L5050 (64.5668, 48.641) -> (63.9572, 48.641)
  line L5051 (66.7817, 51.2877) -> (66.7817, 52.3037)
  line L5052 (58.8772, 53.721) -> (59.4868, 53.721)
  line L5053 (58.882, 53.763) -> (58.882, 52.663)
  line L5054 (66.0959, 50.673) -> (66.0959, 50.0634)
  line L5055 (59.9796, 49.8241) -> (60.5892, 49.8241)
  line L5056 (67.3913, 51.6707) -> (67.3913, 51.9206)
  line L5057 (59.9796, 50.4571) -> (60.5892, 50.4571)
  line L5058 (58.8772, 54.993) -> (59.4868, 54.993)
  line L5059 (66.7865, 52.3457) -> (66.7865, 51.2457)
  line L5060 (65.0379, 50.6682) -> (65.0379, 50.0682)
  line L5061 (67.437, 49.8602) -> (67.437, 50.4698)
  line L5062 (59.4868, 52.705) -> (58.8772, 52.705)
  line L5063 (63.9572, 49.657) -> (64.5668, 49.657)
  line L5064 (58.8772, 54.61) -> (58.8772, 55.626)
  line L5065 (59.482, 52.663) -> (59.482, 53.763)
  line L5066 (58.8772, 53.088) -> (59.4868, 53.088)
  line L5067 (64.562, 49.699) -> (63.962, 49.699)
  line L5068 (67.437, 50.4698) -> (68.453, 50.4698)
  line L5069 (63.9572, 49.657) -> (64.5668, 49.657)
  line L5070 (59.4868, 55.626) -> (59.4868, 54.61)
  line L5071 (67.82, 49.8602) -> (68.07, 49.8602)
  line L5072 (64.562, 48.599) -> (64.562, 49.699)
  line L5073 (68.07, 50.4698) -> (67.82, 50.4698)
  line L5074 (58.8772, 55.626) -> (59.4868, 55.626)
  line L5075 (58.8772, 54.61) -> (58.8772, 55.626)
  line L5076 (63.9572, 48.641) -> (63.9572, 49.657)
  line L5077 (58.8772, 52.705) -> (58.8772, 53.721)
  line L5078 (67.3865, 51.2457) -> (67.3865, 52.3457)
  line L5079 (59.4868, 53.338) -> (58.8772, 53.338)
  line L5080 (61.514, 49.699) -> (60.914, 49.699)
  line L5081 (63.962, 48.599) -> (64.562, 48.599)
  line L5082 (68.453, 50.4698) -> (68.453, 49.8602)
  line L5083 (58.8772, 52.705) -> (58.8772, 53.721)
  line L5084 (66.7817, 52.3037) -> (67.3913, 52.3037)
  line L5085 (67.3913, 51.9206) -> (66.7817, 51.9206)
  line L5086 (63.9572, 48.641) -> (63.9572, 49.657)
  line L5087 (67.437, 50.4698) -> (68.453, 50.4698)
  line L5088 (66.1379, 50.6682) -> (65.0379, 50.6682)
  line L5089 (68.453, 49.8602) -> (67.437, 49.8602)
  line L5090 (67.82, 50.4698) -> (67.82, 49.8602)
  line L5091 (59.4868, 54.993) -> (59.4868, 55.243)
  line L5092 (67.3865, 52.3457) -> (66.7865, 52.3457)
  line L5093 (66.7817, 51.6707) -> (67.3913, 51.6707)
  line L5094 (64.5668, 49.274) -> (63.9572, 49.274)
  line L5095 (58.882, 55.668) -> (58.882, 54.568)
  line L5096 (60.5892, 49.4411) -> (59.9796, 49.4411)
  line L5097 (61.976, 49.1795) -> (61.976, 50.1955)
  line L5098 (67.3913, 51.2877) -> (66.7817, 51.2877)
  line L5099 (74.5998, 50.925) -> (73.9902, 50.925)
  line L5100 (62.946, 48.599) -> (63.546, 48.599)
  line L5101 (62.5808, 49.1375) -> (62.5808, 50.2375)
  line L5102 (62.5856, 49.8124) -> (61.976, 49.8124)
  line L5103 (73.9902, 50.675) -> (74.5998, 50.675)
  line L5104 (62.5856, 50.1955) -> (62.5856, 49.1795)
  line L5105 (63.546, 49.699) -> (62.946, 49.699)
  line L5106 (63.5508, 49.657) -> (63.5508, 48.641)
  line L5107 (66.7817, 51.9206) -> (66.7817, 51.6707)
  line L5108 (60.914, 48.599) -> (61.514, 48.599)
  line L5109 (60.5844, 50.4991) -> (59.9844, 50.4991)
  line L5110 (65.0379, 50.0682) -> (66.1379, 50.0682)
  line L5111 (61.976, 49.1795) -> (61.976, 50.1955)
  line L5112 (59.9796, 49.4411) -> (59.9796, 50.4571)
  line L5113 (61.9808, 50.2375) -> (61.9808, 49.1375)
  line L5114 (61.976, 50.1955) -> (62.5856, 50.1955)
  line L5115 (62.5856, 50.1955) -> (62.5856, 49.1795)
  line L5116 (66.0959, 50.673) -> (66.0959, 50.0634)
  line L5117 (66.7817, 51.2877) -> (66.7817, 52.3037)
  line L5118 (66.7817, 52.3037) -> (67.3913, 52.3037)
  line L5119 (61.5188, 49.657) -> (61.5188, 48.641)
  line L5120 (62.5808, 50.2375) -> (61.9808, 50.2375)
  line L5121 (62.946, 49.699) -> (62.946, 48.599)
  line L5122 (65.0799, 50.0634) -> (65.0799, 50.673)
  line L5123 (63.5508, 48.641) -> (62.9412, 48.641)
  line L5124 (61.976, 49.5625) -> (62.5856, 49.5625)
  line L5125 (65.0799, 50.0634) -> (65.0799, 50.673)
  line L5126 (59.9844, 50.4991) -> (59.9844, 49.3991)
  line L5127 (59.9796, 49.4411) -> (59.9796, 50.4571)
  line L5128 (60.5892, 50.4571) -> (60.5892, 49.4411)
  line L5129 (66.1379, 50.0682) -> (66.1379, 50.6682)
  line L5130 (66.0959, 50.0634) -> (65.0799, 50.0634)
  line L5131 (60.5892, 49.4411) -> (59.9796, 49.4411)
  line L5132 (60.5892, 50.4571) -> (60.5892, 49.4411)
  line L5133 (60.5844, 49.3991) -> (60.5844, 50.4991)
  line L5134 (60.914, 49.699) -> (60.914, 48.599)
  line L5135 (60.5892, 50.0741) -> (59.9796, 50.0741)
  line L5136 (61.976, 50.1955) -> (62.5856, 50.1955)
  line L5137 (63.546, 48.599) -> (63.546, 49.699)
  line L5138 (59.9796, 50.0741) -> (59.9796, 49.8241)
  line L5139 (58.8772, 53.338) -> (58.8772, 53.088)
  line L5140 (73.995, 50.25) -> (74.595, 50.25)
  line L5141 (62.9412, 49.657) -> (63.5508, 49.657)
  line L5142 (65.4629, 50.673) -> (65.4629, 50.0634)
  line L5143 (60.9092, 48.641) -> (60.9092, 49.657)
  line L5144 (61.5188, 49.657) -> (61.5188, 48.641)
  line L5145 (60.5892, 49.8241) -> (60.5892, 50.0741)
  line L5146 (61.514, 48.599) -> (61.514, 49.699)
  line L5147 (62.5856, 49.1795) -> (61.976, 49.1795)
  line L5148 (74.595, 51.35) -> (73.995, 51.35)
  line L5149 (60.9092, 49.657) -> (61.5188, 49.657)
  line L5150 (65.0799, 50.673) -> (66.0959, 50.673)
  line L5151 (60.9092, 49.024) -> (61.5188, 49.024)
  line L5152 (61.5188, 49.274) -> (60.9092, 49.274)
  line L5153 (65.7128, 50.0634) -> (65.7128, 50.673)
  line L5154 (66.7865, 51.2457) -> (67.3865, 51.2457)
  line L5155 (74.595, 50.25) -> (74.595, 51.35)
  line L5156 (60.9092, 48.641) -> (60.9092, 49.657)
  line L5157 (61.5188, 48.641) -> (60.9092, 48.641)
  line L5158 (59.9844, 49.3991) -> (60.5844, 49.3991)
  line L5159 (59.9796, 50.4571) -> (60.5892, 50.4571)
  line L5160 (62.5856, 49.5625) -> (62.5856, 49.8124)
  line L5161 (61.9808, 49.1375) -> (62.5808, 49.1375)
  line L5162 (74.5998, 51.308) -> (74.5998, 50.292)
  line L5163 (27.977, 30.142) -> (29.427, 30.142)
  line L5164 (27.9908, 32.385) -> (27.9908, 30.099)
  line L5165 (27.977, 32.342) -> (27.977, 30.142)
  line L5166 (63.5508, 49.274) -> (62.9412, 49.274)
  line L5167 (82.717, 54.395) -> (81.367, 54.395)
  line L5168 (27.9908, 32.385) -> (27.9908, 30.099)
  line L5169 (82.717, 56.095) -> (81.367, 56.095)
  line L5170 (82.717, 56.095) -> (81.367, 56.095)
  line L5171 (82.7532, 56.388) -> (81.3308, 56.388)
  line L5172 (81.317, 56.345) -> (81.317, 54.145)
  line L5173 (81.3308, 56.388) -> (81.3308, 54.102)
  line L5174 (73.9902, 50.292) -> (73.9902, 51.308)
  line L5175 (60.9092, 49.274) -> (60.9092, 49.024)
  line L5176 (74.5998, 50.292) -> (73.9902, 50.292)
  line L5177 (58.4149, 51.9862) -> (59.4309, 51.9862)
  line L5178 (62.9412, 48.641) -> (62.9412, 49.657)
  line L5179 (29.427, 30.142) -> (29.427, 32.342)
  line L5180 (59.4309, 51.3766) -> (58.4149, 51.3766)
  line L5181 (63.5508, 48.641) -> (62.9412, 48.641)
  line L5182 (74.5998, 50.292) -> (73.9902, 50.292)
  line L5183 (73.9902, 50.292) -> (73.9902, 51.308)
  line L5184 (29.427, 32.342) -> (27.977, 32.342)
  line L5185 (27.9908, 30.099) -> (29.4132, 30.099)
  line L5186 (82.717, 56.095) -> (81.367, 56.095)
  line L5187 (81.3308, 54.102) -> (82.7532, 54.102)
  line L5188 (73.995, 51.35) -> (73.995, 50.25)
  line L5189 (73.9902, 51.308) -> (74.5998, 51.308)
  line L5190 (58.4149, 51.9862) -> (59.4309, 51.9862)
  line L5191 (82.7532, 54.102) -> (82.7532, 56.388)
  line L5192 (82.717, 54.395) -> (81.367, 54.395)
  line L5193 (74.5998, 51.308) -> (74.5998, 50.292)
  line L5194 (81.3308, 54.102) -> (82.7532, 54.102)
  line L5195 (61.976, 49.8124) -> (61.976, 49.5625)
  line L5196 (62.9412, 49.024) -> (63.5508, 49.024)
  line L5197 (61.5188, 48.641) -> (60.9092, 48.641)
  line L5198 (62.9412, 49.274) -> (62.9412, 49.024)
  line L5199 (61.5188, 49.024) -> (61.5188, 49.274)
  line L5200 (60.9092, 49.657) -> (61.5188, 49.657)
  line L5201 (62.9412, 48.641) -> (62.9412, 49.657)
  line L5202 (63.5508, 49.024) -> (63.5508, 49.274)
  line L5203 (62.5856, 49.1795) -> (61.976, 49.1795)
  line L5204 (73.9902, 50.925) -> (73.9902, 50.675)
  line L5205 (59.4309, 51.3766) -> (58.4149, 51.3766)
  line L5206 (62.9412, 49.657) -> (63.5508, 49.657)
  line L5207 (58.4149, 51.3766) -> (58.4149, 51.9862)
  line L5208 (59.4729, 51.3814) -> (59.4729, 51.9814)
  line L5209 (58.3729, 51.3814) -> (59.4729, 51.3814)
  line L5210 (59.4729, 51.9814) -> (58.3729, 51.9814)
  line L5211 (58.3729, 51.9814) -> (58.3729, 51.3814)
  line L5212 (58.4149, 51.3766) -> (58.4149, 51.9862)
  line L5213 (82.717, 54.395) -> (81.367, 54.395)
  line L5214 (59.0479, 51.3766) -> (59.0479, 51.9862)
  line L5215 (82.767, 56.345) -> (81.317, 56.345)
  line L5216 (82.7532, 56.388) -> (81.3308, 56.388)
  line L5217 (59.4309, 51.9862) -> (59.4309, 51.3766)
  line L5218 (59.4309, 51.9862) -> (59.4309, 51.3766)
  line L5219 (58.798, 51.9862) -> (58.798, 51.3766)
  line L5220 (74.5998, 50.675) -> (74.5998, 50.925)
  line L5221 (82.767, 54.145) -> (82.767, 56.345)
  line L5222 (73.9902, 51.308) -> (74.5998, 51.308)
  line L5223 (63.5508, 49.657) -> (63.5508, 48.641)
  line L5224 (72.4408, 1.3208) -> (72.4408, 3.7338)
  line L5225 (29.4132, 30.099) -> (29.4132, 32.385)
  line L5226 (69.112, 1.59) -> (69.112, 3.49)
  line L5227 (81.5086, 59.6011) -> (81.5086, 61.8109)
  line L5228 (79.502, 62.2046) -> (80.518, 62.2046)
  line L5229 (25.9588, 60.071) -> (25.9588, 57.785)
  line L5230 (29.4132, 30.099) -> (29.4132, 32.385)
  line L5231 (72.4408, 3.7338) -> (68.8086, 3.7338)
  line L5232 (81.5086, 59.6011) -> (81.5086, 61.8109)
  line L5233 (68.836, 31.6738) -> (68.836, 31.0642)
  line L5234 (72.112, 1.59) -> (72.112, 3.49)
  line L5235 (81.28, 61.976) -> (78.74, 61.976)
  line L5236 (72.112, 1.59) -> (72.112, 3.49)
  line L5237 (69.112, 1.59) -> (69.112, 3.49)
  line L5238 (68.453, 31.6738) -> (69.469, 31.6738)
  line L5239 (68.8086, 3.7338) -> (68.8086, 1.3208)
  line L5240 (81.28, 59.436) -> (81.28, 61.976)
  line L5241 (79.502, 62.2046) -> (80.518, 62.2046)
  line L5242 (78.5114, 59.6011) -> (78.5114, 61.8109)
  line L5243 (69.469, 31.0642) -> (68.453, 31.0642)
  line L5244 (62.946, 45) -> (62.946, 43.9)
  line L5245 (69.086, 31.0642) -> (69.086, 31.6738)
  line L5246 (78.74, 60.071) -> (79.375, 59.436)
  line L5247 (62.946, 43.9) -> (63.546, 43.9)
  line L5248 (68.453, 31.6738) -> (69.469, 31.6738)
  line L5249 (78.5114, 59.6011) -> (78.5114, 61.8109)
  line L5250 (25.9588, 57.785) -> (27.3812, 57.785)
  line L5251 (28.027, 30.392) -> (29.377, 30.392)
  line L5252 (29.4132, 32.385) -> (27.9908, 32.385)
  line L5253 (25.9588, 60.071) -> (25.9588, 57.785)
  line L5254 (27.395, 60.028) -> (25.945, 60.028)
  line L5255 (81.3308, 56.388) -> (81.3308, 54.102)
  line L5256 (27.345, 59.778) -> (25.995, 59.778)
  line L5257 (27.345, 58.078) -> (25.995, 58.078)
  line L5258 (25.945, 57.828) -> (27.395, 57.828)
  line L5259 (28.027, 32.092) -> (29.377, 32.092)
  line L5260 (62.9412, 43.942) -> (62.9412, 44.958)
  line L5261 (69.511, 31.669) -> (68.411, 31.669)
  line L5262 (59.0479, 51.9862) -> (58.798, 51.9862)
  line L5263 (27.3812, 57.785) -> (27.3812, 60.071)
  line L5264 (27.9908, 30.099) -> (29.4132, 30.099)
  line L5265 (82.7532, 54.102) -> (82.7532, 56.388)
  line L5266 (27.3812, 57.785) -> (27.3812, 60.071)
  line L5267 (27.3812, 60.071) -> (25.9588, 60.071)
  line L5268 (81.317, 54.145) -> (82.767, 54.145)
  line L5269 (58.798, 51.3766) -> (59.0479, 51.3766)
  line L5270 (27.345, 59.778) -> (25.995, 59.778)
  line L5271 (27.3812, 60.071) -> (25.9588, 60.071)
  line L5272 (25.9588, 57.785) -> (27.3812, 57.785)
  line L5273 (28.027, 32.092) -> (29.377, 32.092)
  line L5274 (28.027, 30.392) -> (29.377, 30.392)
  line L5275 (27.345, 58.078) -> (25.995, 58.078)
  line L5276 (68.8086, 1.3208) -> (72.4408, 1.3208)
  line L5277 (28.027, 32.092) -> (29.377, 32.092)
  line L5278 (78.74, 61.976) -> (78.74, 60.071)
  line L5279 (27.345, 59.778) -> (25.995, 59.778)
  line L5280 (69.112, 1.59) -> (69.112, 3.49)
  line L5281 (28.027, 30.392) -> (29.377, 30.392)
  line L5282 (27.395, 57.828) -> (27.395, 60.028)
  line L5283 (72.112, 1.59) -> (72.112, 3.49)
  line L5284 (29.4132, 32.385) -> (27.9908, 32.385)
  line L5285 (25.945, 60.028) -> (25.945, 57.828)
  line L5286 (79.502, 62.2046) -> (80.518, 62.2046)
  line L5287 (27.345, 58.078) -> (25.995, 58.078)
  line L5288 (62.9412, 43.942) -> (62.9412, 44.958)
  line L5289 (63.5508, 44.958) -> (63.5508, 43.942)
  line L5290 (68.836, 31.0642) -> (69.086, 31.0642)
  line L5291 (79.0194, 61.6966) -> (79.0194, 59.7154)
  line L5292 (63.5508, 43.942) -> (62.9412, 43.942)
  line L5293 (63.546, 43.9) -> (63.546, 45)
  line L5294 (69.469, 31.6738) -> (69.469, 31.0642)
  line L5295 (81.0006, 59.7154) -> (81.0006, 61.6966)
  line L5296 (69.469, 31.0642) -> (68.453, 31.0642)
  line L5297 (63.5508, 43.942) -> (62.9412, 43.942)
  line L5298 (69.511, 31.069) -> (69.511, 31.669)
  line L5299 (62.9412, 44.325) -> (63.5508, 44.325)
  line L5300 (79.502, 59.2074) -> (80.518, 59.2074)
  line L5301 (68.411, 31.669) -> (68.411, 31.069)
  line L5302 (79.375, 59.436) -> (81.28, 59.436)
  line L5303 (81.0006, 61.6966) -> (79.0194, 61.6966)
  line L5304 (81.5086, 59.6011) -> (81.5086, 61.8109)
  line L5305 (62.9412, 44.958) -> (63.5508, 44.958)
  line L5306 (63.5508, 44.958) -> (63.5508, 43.942)
  line L5307 (62.9412, 44.958) -> (63.5508, 44.958)
  line L5308 (68.411, 31.069) -> (69.511, 31.069)
  line L5309 (78.5114, 59.6011) -> (78.5114, 61.8109)
  line L5310 (69.469, 31.6738) -> (69.469, 31.0642)
  line L5311 (68.453, 31.0642) -> (68.453, 31.6738)
  line L5312 (79.502, 59.2074) -> (80.518, 59.2074)
  line L5313 (79.0194, 59.7154) -> (81.0006, 59.7154)
  line L5314 (63.5508, 44.325) -> (63.5508, 44.575)
  line L5315 (79.502, 59.2074) -> (80.518, 59.2074)
  line L5316 (63.546, 45) -> (62.946, 45)
  line L5317 (62.9412, 44.575) -> (62.9412, 44.325)
  line L5318 (69.086, 31.6738) -> (68.836, 31.6738)
  line L5319 (63.5508, 44.575) -> (62.9412, 44.575)
  line L5320 (68.453, 31.0642) -> (68.453, 31.6738)
  line L5321 (81.542, 38.5135) -> (81.542, 38.9885)
  line L5322 (75.4, 16.526) -> (77, 16.526)
  line L5323 (75.049, 38.8615) -> (75.049, 38.3865)
  line L5324 (75.9, 16.876) -> (75.1, 16.876)
  line L5325 (74.049, 40.8615) -> (74.049, 40.3865)
  arc A2942 (73.549, 40.6748) -> (73.549, 40.5732) centre (73.549, 40.624) ccw
  line L5326 (73.3115, 39.124) -> (73.7865, 39.124)
  arc A2943 (75.5034, 41.1539) -> (75.5034, 40.9229) centre (75.5034, 41.0384) ccw